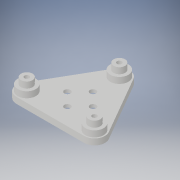
# Autodesk Inventor part: PlanetaryHolderTop
Saved by Autodesk Inventor 2018.3 (Build 223284000, 284)
## iProperties
Created: 2018-07-08
Part Number: PlanetaryHolderTop
Material: Generisch
Document SubType Name: Modeling
Designer: JochenAlt
Density: 1 g/cm^3
Appearance: Vorgabe
Author: JochenAlt
Autodesk Inventor part; units mm, degrees
ref_plane "YZ Plane" through (0, 0, 0) normal (1, 0, 0) x (0, 1, 0)
ref_plane "XZ Plane" through (0, 0, 0) normal (0, 1, 0) x (-1, 0, 0)
ref_plane "XY Plane" through (0, 0, 0) normal (0, 0, 1) x (1, 0, 0)
sketch "Skizze1" plane through (0, 0, 0) normal (0, 0, 1) x (1, 0, 0)
  circle A0 centre (0, 0) radius 19.4 construction
  circle A1 centre (0, 0) radius 9.75
  circle A2 centre (0, 19.4) radius 1.15
  line L0 (0, 0) -> (-16.8009, -9.7) construction
  line L1 (0, 34.057) -> (0, -28.3095) construction
  line L2 (-32.8873, 0) -> (32.8873, 0) construction
  circle A3 centre (0, 0) radius 6.35 construction
  circle A4 centre (0, 6.35) radius 1.5
  circle A5 centre (0, -6.35) radius 1.5
  circle A6 centre (6.35, 0) radius 1.5
  circle A7 centre (-6.35, 0) radius 1.5
  arc A8 (0, 24.55) -> (-4.46, 21.975) centre (0, 19.4) ccw
  circle A9 centre (16.8009, -9.7) radius 1.15
  arc A10 (16.8009, -14.85) -> (21.2609, -7.125) centre (16.8009, -9.7) ccw
  circle A11 centre (-16.8009, -9.7) radius 1.15
  arc A12 (-21.2609, -7.125) -> (-16.8009, -14.85) centre (-16.8009, -9.7) ccw
  circle A13 centre (0, 19.4) radius 2.85
  circle A14 centre (16.8009, -9.7) radius 2.85
  circle A15 centre (-16.8009, -9.7) radius 2.85
  circle A16 centre (0, 19.4) radius 4.5
  circle A17 centre (16.8009, -9.7) radius 4.5
  circle A18 centre (-16.8009, -9.7) radius 4.5
  line L3 (-4.46, 21.975) -> (-21.2609, -7.125)
  line L4 (-16.8009, -14.85) -> (16.8009, -14.85)
  line L5 (4.46, 21.975) -> (21.2609, -7.125)
  arc A19 (4.46, 21.975) -> (0, 24.55) centre (0, 19.4) ccw
  circle A20 centre (0, 19.4) radius 2.2 construction
  line L6 (1.2702, 21.6) -> (2.5403, 19.4)
  line L7 (2.5403, 19.4) -> (1.2702, 17.2)
  line L8 (1.2702, 17.2) -> (-1.2702, 17.2)
  line L9 (-1.2702, 17.2) -> (-2.5403, 19.4)
  line L10 (-2.5403, 19.4) -> (-1.2702, 21.6)
  line L11 (-1.2702, 21.6) -> (1.2702, 21.6)
  circle A21 centre (-16.8009, -9.7) radius 2.2 construction
  circle A22 centre (16.8009, -9.7) radius 2.2 construction
  line L12 (-18.0695, -11.9009) -> (-19.3412, -9.7018)
  line L13 (-19.3412, -9.7018) -> (-18.0726, -7.5009)
  line L14 (-18.0726, -7.5009) -> (-15.5322, -7.4991)
  line L15 (-15.5322, -7.4991) -> (-14.2606, -9.6982)
  line L16 (-14.2606, -9.6982) -> (-15.5292, -11.8991)
  line L17 (-15.5292, -11.8991) -> (-18.0695, -11.9009)
  line L18 (15.865, -12.0617) -> (14.2877, -10.0703)
  line L19 (14.2877, -10.0703) -> (15.2236, -7.7087)
  line L20 (15.2236, -7.7087) -> (17.7368, -7.3383)
  line L21 (17.7368, -7.3383) -> (19.3141, -9.3297)
  line L22 (19.3141, -9.3297) -> (18.3782, -11.6913)
  line L23 (18.3782, -11.6913) -> (15.865, -12.0617)
  point P0 (0, 21.6)
  point P1 (-16.8009, -9.7)
  point P2 (-16.7994, -11.9)
  point P3 (17.1216, -11.8765)
  dimension "d31" = 4.4
  dimension "d0" = 38.8
  dimension "d1" = 2.3
  dimension "d2" = 30
  dimension "d3" = 19.5
  dimension "d4" = 12.7
  dimension "d5" = 3
  dimension "d8" = 4
  dimension "d26" = 5.7
  dimension "d30" = 9
  constraints: 44 end point, 20 centre point, 19 coincident, 16 point on circle, 12 equal radius, 7 point on line, 6 tangent, 3 midpoint, 1 concentric, 1 symmetric about line, 1 vertical alignment, 48 other
  measures "d0" diameter of A0
  measures "d1" diameter of A2
  measures "d2" angle of L0 L2
  measures "d3" diameter of A1
  measures "d4" diameter of A3
  measures "d5" diameter of A4
  measures "d8" radial gap between concentric circles of A2 A8
  measures "d26" diameter of A13
  measures "d30" diameter of A16
extrude "Extrusion1" add sketch "Skizze1" along normal blind 3 contours A1 | A19 L5 A10 L4 A12 L3 A8 | A13 | A14 | A15 | A16 | A17 | A18 | L6 L7 L8 L9 L10 L11 | L12 L13 L14 L15 L16 L17 | L18 L19 L20 L21 L22 L23
extrude "Extrusion3" cut sketch "Skizze1" along normal blind 1.5 contours A1
extrude "Extrusion4" add sketch "Skizze1" along normal blind 3 from surface at 3 contours A13 | A14 | A15 | A16 | A17 | A18 | L6 L7 L8 L9 L10 L11 | L12 L13 L14 L15 L16 L17 | L18 L19 L20 L21 L22 L23
extrude "Extrusion6" add sketch "Skizze1" along normal blind 3 from surface at 6 contours A13 | A14 | A15 | L6 L7 L8 L9 L10 L11 | L12 L13 L14 L15 L16 L17 | L18 L19 L20 L21 L22 L23
extrude "Extrusion8" cut sketch "Skizze1" along normal blind 1.5 contours L6 L7 L8 L9 L10 L11 | L12 L13 L14 L15 L16 L17 | L18 L19 L20 L21 L22 L23
